Autodesk Inventor part; units mm, degrees
(part 3 of 3)
  spline S181 degree 2 poles (565.5506, -57.2741) (560.0725, -57.2741) (552.7403, -57.9484) (549.8748, -59.044) knots 0 0 0 1 2 2 2
  spline S182 degree 2 poles (549.8748, -59.044) (547.1779, -60.0553) (544.2702, -63.8058) (544.2702, -66.8398) knots 0 0 0 1 2 2 2
  spline S183 degree 2 poles (544.2702, -66.8398) (544.2702, -69.7053) (547.0093, -73.4557) (549.7484, -74.5092) knots 0 0 0 1 2 2 2
  spline S184 degree 2 poles (556.4485, -145.3033) (552.4453, -145.3033) (545.6608, -142.6485) (543.3853, -140.4152) knots 0 0 0 1 2 2 2
  spline S185 degree 2 poles (543.3853, -140.4152) (540.9834, -138.0975) (538.4971, -132.2822) (538.4971, -128.7847) knots 0 0 0 1 2 2 2
  spline S186 degree 2 poles (538.4971, -128.7847) (538.4971, -125.2871) (540.857, -119.514) (543.2168, -117.3228) knots 0 0 0 1 2 2 2
  spline S187 degree 2 poles (543.2168, -117.3228) (546.0401, -114.6258) (555.5215, -111.5918) (562.4323, -111.5918) knots 0 0 0 1 2 2 2
  spline S188 degree 2 poles (562.4323, -111.5918) (569.2168, -111.5918) (580.1309, -114.373) (584.1762, -117.2806) knots 0 0 0 1 2 2 2
  spline S189 degree 2 poles (584.1762, -117.2806) (588.1373, -120.104) (592.562, -129.0375) (592.562, -134.8949) knots 0 0 0 1 2 2 2
  spline S190 degree 2 poles (592.562, -134.8949) (592.562, -136.6226) (592.2249, -139.6566) (591.8456, -140.7944) knots 0 0 0 1 2 2 2
  line L106 (591.8456, -140.7944) -> (585.1454, -140.7944)
  line L107 (585.1454, -140.7944) -> (585.1454, -140.4994)
  spline S191 degree 2 poles (585.1454, -140.4994) (585.6511, -139.5302) (586.536, -135.9905) (586.536, -133.9678) knots 0 0 0 1 2 2 2
  spline S192 degree 2 poles (586.536, -133.9678) (586.536, -127.4784) (577.7711, -119.514) (569.1746, -118.7555) knots 0 0 0 1 2 2 2
  spline S193 degree 2 poles (569.1746, -118.7555) (570.9023, -121.2417) (572.7986, -126.467) (572.7986, -129.5853) knots 0 0 0 1 2 2 2
  spline S194 degree 2 poles (572.7986, -129.5853) (572.7986, -132.6194) (571.5766, -137.1704) (569.7224, -139.6566) knots 0 0 0 1 2 2 2
  spline S195 degree 2 poles (569.7224, -139.6566) (567.5733, -142.5221) (560.9153, -145.3033) (556.4485, -145.3033) knots 0 0 0 1 2 2 2
  spline S196 degree 2 poles (556.1535, -138.2239) (559.3561, -138.2239) (563.6965, -136.5383) (565.2135, -134.6842) knots 0 0 0 1 2 2 2
  spline S197 degree 2 poles (565.2135, -134.6842) (566.3091, -133.2936) (567.0255, -129.8382) (567.0255, -128.0262) knots 0 0 0 1 2 2 2
  spline S198 degree 2 poles (567.0255, -128.0262) (567.0255, -125.5821) (565.5506, -120.9889) (564.16, -118.7555) knots 0 0 0 1 2 2 2
  spline S199 degree 2 poles (564.16, -118.7555) (563.4015, -118.7134) (561.9688, -118.6291) (560.8732, -118.6291) knots 0 0 0 1 2 2 2
  spline S200 degree 2 poles (560.8732, -118.6291) (555.4793, -118.6291) (548.8634, -120.7361) (547.1357, -122.3374) knots 0 0 0 1 2 2 2
  spline S201 degree 2 poles (547.1357, -122.3374) (545.4923, -123.8122) (544.186, -127.0148) (544.186, -128.8268) knots 0 0 0 1 2 2 2
  spline S202 degree 2 poles (544.186, -128.8268) (544.186, -133.0408) (550.1698, -138.2239) (556.1535, -138.2239) knots 0 0 0 1 2 2 2
  spline S203 degree 2 poles (565.5928, -183.8187) (551.6025, -183.8187) (538.4971, -175.6858) (538.4971, -167.2158) knots 0 0 0 1 2 2 2
  spline S204 degree 2 poles (538.4971, -167.2158) (538.4971, -158.6194) (551.8553, -150.5707) (565.5506, -150.5707) knots 0 0 0 1 2 2 2
  spline S205 degree 2 poles (565.5506, -150.5707) (579.6252, -150.5707) (592.6463, -158.7036) (592.6463, -167.2158) knots 0 0 0 1 2 2 2
  spline S206 degree 2 poles (592.6463, -167.2158) (592.6463, -175.7701) (579.1617, -183.8187) (565.5928, -183.8187) knots 0 0 0 1 2 2 2
  spline S207 degree 2 poles (549.7484, -174.8852) (552.3189, -175.8965) (560.2411, -176.7393) (565.5928, -176.7393) knots 0 0 0 1 2 2 2
  spline S208 degree 2 poles (565.5928, -176.7393) (570.9445, -176.7393) (578.8245, -175.8965) (581.4793, -174.843) knots 0 0 0 1 2 2 2
  spline S209 degree 2 poles (581.4793, -174.843) (584.1341, -173.7895) (586.8732, -170.1234) (586.8732, -167.2158) knots 0 0 0 1 2 2 2
  spline S210 degree 2 poles (586.8732, -167.2158) (586.8732, -164.3082) (584.1341, -160.5578) (581.395, -159.4622) knots 0 0 0 1 2 2 2
  spline S211 degree 2 poles (581.395, -159.4622) (578.7403, -158.4087) (570.6495, -157.6502) (565.5506, -157.6502) knots 0 0 0 1 2 2 2
  spline S212 degree 2 poles (565.5506, -157.6502) (560.0725, -157.6502) (552.7403, -158.3244) (549.8748, -159.42) knots 0 0 0 1 2 2 2
  spline S213 degree 2 poles (549.8748, -159.42) (547.1779, -160.4314) (544.2702, -164.1818) (544.2702, -167.2158) knots 0 0 0 1 2 2 2
  spline S214 degree 2 poles (544.2702, -167.2158) (544.2702, -170.0813) (547.0093, -173.8317) (549.7484, -174.8852) knots 0 0 0 1 2 2 2
  line L108 (583.797, -245.4686) -> (539.5928, -222.9662)
  line L109 (539.5928, -222.9662) -> (539.5928, -215.5497)
  line L110 (539.5928, -215.5497) -> (585.4826, -239.3163)
  line L111 (585.4826, -239.3163) -> (585.4826, -212.4735)
  line L112 (585.4826, -212.4735) -> (591.5928, -212.4735)
  line L113 (591.5928, -212.4735) -> (591.5928, -245.4686)
  line L114 (591.5928, -245.4686) -> (583.797, -245.4686)
  spline S215 degree 2 poles (565.5928, -284.1947) (551.6025, -284.1947) (538.4971, -276.0618) (538.4971, -267.5918) knots 0 0 0 1 2 2 2
  spline S216 degree 2 poles (538.4971, -267.5918) (538.4971, -258.9954) (551.8553, -250.9468) (565.5506, -250.9468) knots 0 0 0 1 2 2 2
  spline S217 degree 2 poles (565.5506, -250.9468) (579.6252, -250.9468) (592.6463, -259.0797) (592.6463, -267.5918) knots 0 0 0 1 2 2 2
  spline S218 degree 2 poles (592.6463, -267.5918) (592.6463, -276.1461) (579.1617, -284.1947) (565.5928, -284.1947) knots 0 0 0 1 2 2 2
  spline S219 degree 2 poles (549.7484, -275.2612) (552.3189, -276.2725) (560.2411, -277.1153) (565.5928, -277.1153) knots 0 0 0 1 2 2 2
  spline S220 degree 2 poles (565.5928, -277.1153) (570.9445, -277.1153) (578.8245, -276.2725) (581.4793, -275.219) knots 0 0 0 1 2 2 2
  spline S221 degree 2 poles (581.4793, -275.219) (584.1341, -274.1656) (586.8732, -270.4994) (586.8732, -267.5918) knots 0 0 0 1 2 2 2
  spline S222 degree 2 poles (586.8732, -267.5918) (586.8732, -264.6842) (584.1341, -260.9338) (581.395, -259.8382) knots 0 0 0 1 2 2 2
  spline S223 degree 2 poles (581.395, -259.8382) (578.7403, -258.7847) (570.6495, -258.0262) (565.5506, -258.0262) knots 0 0 0 1 2 2 2
  spline S224 degree 2 poles (565.5506, -258.0262) (560.0725, -258.0262) (552.7403, -258.7004) (549.8748, -259.796) knots 0 0 0 1 2 2 2
  spline S225 degree 2 poles (549.8748, -259.796) (547.1779, -260.8074) (544.2702, -264.5578) (544.2702, -267.5918) knots 0 0 0 1 2 2 2
  spline S226 degree 2 poles (544.2702, -267.5918) (544.2702, -270.4573) (547.0093, -274.2077) (549.7484, -275.2612) knots 0 0 0 1 2 2 2
  spline S227 degree 2 poles (538.4129, -328.9046) (538.4129, -325.0278) (540.7305, -318.6647) (542.8796, -316.4314) knots 0 0 0 1 2 2 2
  spline S228 degree 2 poles (542.8796, -316.4314) (544.9866, -314.2401) (550.7176, -311.9646) (553.9623, -311.9646) knots 0 0 0 1 2 2 2
  spline S229 degree 2 poles (553.9623, -311.9646) (558.1762, -311.9646) (565.2557, -316.4735) (567.3626, -320.7717) knots 0 0 0 1 2 2 2
  line L115 (567.3626, -320.7717) -> (567.5733, -320.7717)
  spline S230 degree 2 poles (567.5733, -320.7717) (569.8067, -316.937) (575.1163, -313.2288) (579.0774, -313.2288) knots 0 0 0 1 2 2 2
  spline S231 degree 2 poles (579.0774, -313.2288) (584.9347, -313.2288) (592.7727, -322.078) (592.7727, -328.9046) knots 0 0 0 1 2 2 2
  spline S232 degree 2 poles (592.7727, -328.9046) (592.7727, -335.984) (585.3561, -344.5383) (579.5409, -344.5383) knots 0 0 0 1 2 2 2
  spline S233 degree 2 poles (579.5409, -344.5383) (576.0433, -344.5383) (569.2168, -340.4508) (567.2783, -336.6161) knots 0 0 0 1 2 2 2
  line L116 (567.2783, -336.6161) -> (567.0676, -336.6161)
  spline S234 degree 2 poles (567.0676, -336.6161) (564.9607, -341.1672) (558.8926, -345.8446) (554.0887, -345.8446) knots 0 0 0 1 2 2 2
  spline S235 degree 2 poles (554.0887, -345.8446) (547.4307, -345.8446) (538.4129, -336.1526) (538.4129, -328.9046) knots 0 0 0 1 2 2 2
  spline S236 degree 2 poles (553.4145, -338.6809) (556.6171, -338.6809) (560.4096, -336.1526) (562.348, -332.5707) knots 0 0 0 1 2 2 2
  spline S237 degree 2 poles (562.348, -332.5707) (563.0223, -331.3908) (564.5814, -327.4297) (565.5928, -324.9435) knots 0 0 0 1 2 2 2
  spline S238 degree 2 poles (565.5928, -324.9435) (563.6965, -322.078) (558.0498, -319.0019) (554.468, -319.0019) knots 0 0 0 1 2 2 2
  spline S239 degree 2 poles (554.468, -319.0019) (549.7484, -319.0019) (543.596, -324.6907) (543.596, -328.9889) knots 0 0 0 1 2 2 2
  spline S240 degree 2 poles (543.596, -328.9889) (543.596, -333.3714) (548.8634, -338.6809) (553.4145, -338.6809) knots 0 0 0 1 2 2 2
  spline S241 degree 2 poles (579.4566, -337.7117) (582.9542, -337.7117) (587.6317, -333.0343) (587.6317, -328.8625) knots 0 0 0 1 2 2 2
  spline S242 degree 2 poles (587.6317, -328.8625) (587.6317, -325.0699) (583.4599, -320.2239) (579.878, -320.2239) knots 0 0 0 1 2 2 2
  spline S243 degree 2 poles (579.878, -320.2239) (577.3075, -320.2239) (573.7257, -322.7101) (572.2929, -325.1963) knots 0 0 0 1 2 2 2
  spline S244 degree 2 poles (572.2929, -325.1963) (571.703, -326.2498) (569.6382, -330.7166) (569.0482, -332.5286) knots 0 0 0 1 2 2 2
  spline S245 degree 2 poles (569.0482, -332.5286) (571.3659, -335.5626) (576.2962, -337.7117) (579.4566, -337.7117) knots 0 0 0 1 2 2 2
  spline S246 degree 2 poles (565.5928, -384.5707) (551.6025, -384.5707) (538.4971, -376.4378) (538.4971, -367.9678) knots 0 0 0 1 2 2 2
  spline S247 degree 2 poles (538.4971, -367.9678) (538.4971, -359.3714) (551.8553, -351.3228) (565.5506, -351.3228) knots 0 0 0 1 2 2 2
  spline S248 degree 2 poles (565.5506, -351.3228) (579.6252, -351.3228) (592.6463, -359.4557) (592.6463, -367.9678) knots 0 0 0 1 2 2 2
  spline S249 degree 2 poles (592.6463, -367.9678) (592.6463, -376.5221) (579.1617, -384.5707) (565.5928, -384.5707) knots 0 0 0 1 2 2 2
  spline S250 degree 2 poles (549.7484, -375.6372) (552.3189, -376.6485) (560.2411, -377.4913) (565.5928, -377.4913) knots 0 0 0 1 2 2 2
  spline S251 degree 2 poles (565.5928, -377.4913) (570.9445, -377.4913) (578.8245, -376.6485) (581.4793, -375.595) knots 0 0 0 1 2 2 2
  spline S252 degree 2 poles (581.4793, -375.595) (584.1341, -374.5416) (586.8732, -370.8754) (586.8732, -367.9678) knots 0 0 0 1 2 2 2
  spline S253 degree 2 poles (586.8732, -367.9678) (586.8732, -365.0602) (584.1341, -361.3098) (581.395, -360.2142) knots 0 0 0 1 2 2 2
  spline S254 degree 2 poles (581.395, -360.2142) (578.7403, -359.1607) (570.6495, -358.4022) (565.5506, -358.4022) knots 0 0 0 1 2 2 2
  spline S255 degree 2 poles (565.5506, -358.4022) (560.0725, -358.4022) (552.7403, -359.0764) (549.8748, -360.172) knots 0 0 0 1 2 2 2
  spline S256 degree 2 poles (549.8748, -360.172) (547.1779, -361.1834) (544.2702, -364.9338) (544.2702, -367.9678) knots 0 0 0 1 2 2 2
  spline S257 degree 2 poles (544.2702, -367.9678) (544.2702, -370.8333) (547.0093, -374.5837) (549.7484, -375.6372) knots 0 0 0 1 2 2 2
  spline S258 degree 2 poles (574.6949, -412.1299) (578.6981, -412.1299) (585.3561, -414.7425) (587.7581, -417.0181) knots 0 0 0 1 2 2 2
  spline S259 degree 2 poles (587.7581, -417.0181) (590.0758, -419.1672) (592.6463, -425.4459) (592.6463, -428.6485) knots 0 0 0 1 2 2 2
  spline S260 degree 2 poles (592.6463, -428.6485) (592.6463, -432.2304) (590.2443, -438.0456) (587.9688, -440.1947) knots 0 0 0 1 2 2 2
  spline S261 degree 2 poles (587.9688, -440.1947) (585.1033, -442.8916) (575.8326, -445.8414) (568.7111, -445.8414) knots 0 0 0 1 2 2 2
  spline S262 degree 2 poles (568.7111, -445.8414) (562.2638, -445.8414) (550.7176, -442.9338) (546.8829, -440.1104) knots 0 0 0 1 2 2 2
  spline S263 degree 2 poles (546.8829, -440.1104) (542.8375, -437.1185) (538.5814, -428.6907) (538.5814, -422.5383) knots 0 0 0 1 2 2 2
  spline S264 degree 2 poles (538.5814, -422.5383) (538.5814, -421.1477) (538.8764, -417.9873) (539.2978, -416.6388) knots 0 0 0 1 2 2 2
  line L117 (539.2978, -416.6388) -> (545.998, -416.6388)
  line L118 (545.998, -416.6388) -> (545.998, -416.9759)
  spline S265 degree 2 poles (545.998, -416.9759) (545.4923, -417.8608) (544.6074, -421.5691) (544.6074, -423.4654) knots 0 0 0 1 2 2 2
  spline S266 degree 2 poles (544.6074, -423.4654) (544.6074, -430.292) (553.6252, -438.0877) (561.9688, -438.6356) knots 0 0 0 1 2 2 2
  spline S267 degree 2 poles (561.9688, -438.6356) (560.0725, -435.8544) (558.3448, -430.7976) (558.3448, -427.8057) knots 0 0 0 1 2 2 2
  spline S268 degree 2 poles (558.3448, -427.8057) (558.3448, -424.9403) (559.609, -420.1785) (561.421, -417.7766) knots 0 0 0 1 2 2 2
  spline S269 degree 2 poles (561.421, -417.7766) (563.5701, -414.9954) (570.1017, -412.1299) (574.6949, -412.1299) knots 0 0 0 1 2 2 2
  spline S270 degree 2 poles (570.2702, -438.8041) (575.5377, -438.8041) (582.1957, -436.8657) (584.0077, -435.138) knots 0 0 0 1 2 2 2
  spline S271 degree 2 poles (584.0077, -435.138) (585.6933, -433.621) (586.9574, -430.4605) (586.9574, -428.6064) knots 0 0 0 1 2 2 2
  spline S272 degree 2 poles (586.9574, -428.6064) (586.9574, -424.3082) (580.8051, -419.2093) (574.9899, -419.2093) knots 0 0 0 1 2 2 2
  spline S273 degree 2 poles (574.9899, -419.2093) (571.703, -419.2093) (567.4469, -420.8949) (565.9299, -422.749) knots 0 0 0 1 2 2 2
  spline S274 degree 2 poles (565.9299, -422.749) (564.8343, -424.0975) (564.1179, -427.4265) (564.1179, -429.3649) knots 0 0 0 1 2 2 2
  spline S275 degree 2 poles (564.1179, -429.3649) (564.1179, -431.5983) (565.677, -436.7393) (566.9834, -438.6777) knots 0 0 0 1 2 2 2
  spline S276 degree 2 poles (566.9834, -438.6777) (567.489, -438.7198) (569.2168, -438.8041) (570.2702, -438.8041) knots 0 0 0 1 2 2 2
  spline S277 degree 2 poles (565.5928, -484.9467) (551.6025, -484.9467) (538.4971, -476.8138) (538.4971, -468.3438) knots 0 0 0 1 2 2 2
  spline S278 degree 2 poles (538.4971, -468.3438) (538.4971, -459.7474) (551.8553, -451.6988) (565.5506, -451.6988) knots 0 0 0 1 2 2 2
  spline S279 degree 2 poles (565.5506, -451.6988) (579.6252, -451.6988) (592.6463, -459.8317) (592.6463, -468.3438) knots 0 0 0 1 2 2 2
  spline S280 degree 2 poles (592.6463, -468.3438) (592.6463, -476.8981) (579.1617, -484.9467) (565.5928, -484.9467) knots 0 0 0 1 2 2 2
  spline S281 degree 2 poles (549.7484, -476.0132) (552.3189, -477.0245) (560.2411, -477.8673) (565.5928, -477.8673) knots 0 0 0 1 2 2 2
  spline S282 degree 2 poles (565.5928, -477.8673) (570.9445, -477.8673) (578.8245, -477.0245) (581.4793, -475.9711) knots 0 0 0 1 2 2 2
  spline S283 degree 2 poles (581.4793, -475.9711) (584.1341, -474.9176) (586.8732, -471.2514) (586.8732, -468.3438) knots 0 0 0 1 2 2 2
  spline S284 degree 2 poles (586.8732, -468.3438) (586.8732, -465.4362) (584.1341, -461.6858) (581.395, -460.5902) knots 0 0 0 1 2 2 2
  spline S285 degree 2 poles (581.395, -460.5902) (578.7403, -459.5367) (570.6495, -458.7782) (565.5506, -458.7782) knots 0 0 0 1 2 2 2
  spline S286 degree 2 poles (565.5506, -458.7782) (560.0725, -458.7782) (552.7403, -459.4524) (549.8748, -460.548) knots 0 0 0 1 2 2 2
  spline S287 degree 2 poles (549.8748, -460.548) (547.1779, -461.5594) (544.2702, -465.3098) (544.2702, -468.3438) knots 0 0 0 1 2 2 2
  spline S288 degree 2 poles (544.2702, -468.3438) (544.2702, -471.2093) (547.0093, -474.9597) (549.7484, -476.0132) knots 0 0 0 1 2 2 2
  spline S289 degree 2 poles (441.8635, 560.8836) (441.8635, 574.8739) (449.9964, 587.9792) (458.4664, 587.9792) knots 0 0 0 1 2 2 2
  spline S290 degree 2 poles (458.4664, 587.9792) (467.0628, 587.9792) (475.1114, 574.6211) (475.1114, 560.9258) knots 0 0 0 1 2 2 2
  spline S291 degree 2 poles (475.1114, 560.9258) (475.1114, 546.8512) (466.9785, 533.8301) (458.4664, 533.8301) knots 0 0 0 1 2 2 2
  spline S292 degree 2 poles (458.4664, 533.8301) (449.9121, 533.8301) (441.8635, 547.3147) (441.8635, 560.8836) knots 0 0 0 1 2 2 2
  spline S293 degree 2 poles (450.797, 576.728) (449.7857, 574.1575) (448.9429, 566.2353) (448.9429, 560.8836) knots 0 0 0 1 2 2 2
  spline S294 degree 2 poles (448.9429, 560.8836) (448.9429, 555.5319) (449.7857, 547.6519) (450.8392, 544.9971) knots 0 0 0 1 2 2 2
  spline S295 degree 2 poles (450.8392, 544.9971) (451.8926, 542.3423) (455.5588, 539.6032) (458.4664, 539.6032) knots 0 0 0 1 2 2 2
  spline S296 degree 2 poles (458.4664, 539.6032) (461.374, 539.6032) (465.1244, 542.3423) (466.22, 545.0814) knots 0 0 0 1 2 2 2
  spline S297 degree 2 poles (466.22, 545.0814) (467.2735, 547.7361) (468.032, 555.8269) (468.032, 560.9258) knots 0 0 0 1 2 2 2
  spline S298 degree 2 poles (468.032, 560.9258) (468.032, 566.4039) (467.3578, 573.7361) (466.2622, 576.6016) knots 0 0 0 1 2 2 2
  spline S299 degree 2 poles (466.2622, 576.6016) (465.2508, 579.2985) (461.5004, 582.2061) (458.4664, 582.2061) knots 0 0 0 1 2 2 2
  spline S300 degree 2 poles (458.4664, 582.2061) (455.6009, 582.2061) (451.8505, 579.4671) (450.797, 576.728) knots 0 0 0 1 2 2 2
  line L119 (361.0823, 586.8836) -> (386.4502, 586.8836)
  line L120 (386.4502, 586.8836) -> (386.4502, 581.5741)
  line L121 (386.4502, 581.5741) -> (377.011, 581.5741)
  line L122 (377.011, 581.5741) -> (377.011, 546.7248)
  line L123 (377.011, 546.7248) -> (386.4502, 546.7248)
  line L124 (386.4502, 546.7248) -> (386.4502, 541.963)
  spline S301 degree 2 poles (386.4502, 541.963) (381.0985, 541.963) (376.0417, 538.929) (375.7046, 534.7151) knots 0 0 0 1 2 2 2
  line L125 (375.7046, 534.7151) -> (370.3108, 534.7151)
  line L126 (370.3108, 534.7151) -> (370.3108, 581.5741)
  line L127 (370.3108, 581.5741) -> (361.0823, 581.5741)
  line L128 (361.0823, 581.5741) -> (361.0823, 586.8836)
  spline S302 degree 2 poles (319.1536, 560.8836) (319.1536, 574.8739) (327.2865, 587.9792) (335.7565, 587.9792) knots 0 0 0 1 2 2 2
  spline S303 degree 2 poles (335.7565, 587.9792) (344.3529, 587.9792) (352.4016, 574.6211) (352.4016, 560.9258) knots 0 0 0 1 2 2 2
  spline S304 degree 2 poles (352.4016, 560.9258) (352.4016, 546.8512) (344.2687, 533.8301) (335.7565, 533.8301) knots 0 0 0 1 2 2 2
  spline S305 degree 2 poles (335.7565, 533.8301) (327.2022, 533.8301) (319.1536, 547.3147) (319.1536, 560.8836) knots 0 0 0 1 2 2 2
  spline S306 degree 2 poles (328.0871, 576.728) (327.0758, 574.1575) (326.233, 566.2353) (326.233, 560.8836) knots 0 0 0 1 2 2 2
  spline S307 degree 2 poles (326.233, 560.8836) (326.233, 555.5319) (327.0758, 547.6519) (328.1293, 544.9971) knots 0 0 0 1 2 2 2
  spline S308 degree 2 poles (328.1293, 544.9971) (329.1828, 542.3423) (332.8489, 539.6032) (335.7565, 539.6032) knots 0 0 0 1 2 2 2
  spline S309 degree 2 poles (335.7565, 539.6032) (338.6641, 539.6032) (342.4145, 542.3423) (343.5101, 545.0814) knots 0 0 0 1 2 2 2
  spline S310 degree 2 poles (343.5101, 545.0814) (344.5636, 547.7361) (345.3221, 555.8269) (345.3221, 560.9258) knots 0 0 0 1 2 2 2
  spline S311 degree 2 poles (345.3221, 560.9258) (345.3221, 566.4039) (344.6479, 573.7361) (343.5523, 576.6016) knots 0 0 0 1 2 2 2
  spline S312 degree 2 poles (343.5523, 576.6016) (342.5409, 579.2985) (338.7905, 582.2061) (335.7565, 582.2061) knots 0 0 0 1 2 2 2
  spline S313 degree 2 poles (335.7565, 582.2061) (332.891, 582.2061) (329.1406, 579.4671) (328.0871, 576.728) knots 0 0 0 1 2 2 2
  line L129 (258.0936, 586.8836) -> (290.1617, 586.8836)
  line L130 (290.1617, 586.8836) -> (290.1617, 579.5092)
  spline S314 degree 2 poles (290.1617, 579.5092) (286.7063, 576.2645) (280.5539, 570.2386) (277.6042, 566.9938) knots 0 0 0 1 2 2 2
  spline S315 degree 2 poles (277.6042, 566.9938) (271.6625, 560.4622) (267.3221, 552.6243) (267.3221, 548.4525) knots 0 0 0 1 2 2 2
  spline S316 degree 2 poles (267.3221, 548.4525) (267.3221, 546.2613) (268.6706, 542.9744) (269.8926, 541.9209) knots 0 0 0 1 2 2 2
  spline S317 degree 2 poles (269.8926, 541.9209) (271.1147, 540.8674) (274.3173, 539.8139) (276.2557, 539.8139) knots 0 0 0 1 2 2 2
  spline S318 degree 2 poles (276.2557, 539.8139) (278.1098, 539.8139) (281.9024, 540.741) (283.6301, 541.4574) knots 0 0 0 1 2 2 2
  spline S319 degree 2 poles (283.6301, 541.4574) (285.105, 542.0473) (287.844, 543.7329) (288.6868, 544.3228) knots 0 0 0 1 2 2 2
  line L131 (288.6868, 544.3228) -> (289.0661, 544.3228)
  line L132 (289.0661, 544.3228) -> (289.0661, 536.9063)
  spline S320 degree 2 poles (289.0661, 536.9063) (286.917, 535.8528) (279.2054, 533.788) (275.75, 533.788) knots 0 0 0 1 2 2 2
  spline S321 degree 2 poles (275.75, 533.788) (268.4599, 533.788) (260.2427, 541.4995) (260.2427, 548.0733) knots 0 0 0 1 2 2 2
  spline S322 degree 2 poles (260.2427, 548.0733) (260.2427, 551.1494) (261.6755, 556.2904) (262.9396, 558.4817) knots 0 0 0 1 2 2 2
  spline S323 degree 2 poles (262.9396, 558.4817) (264.2038, 560.7572) (267.87, 565.224) (269.8926, 567.3731) knots 0 0 0 1 2 2 2
  spline S324 degree 2 poles (269.8926, 567.3731) (273.1795, 570.9549) (281.2281, 578.6243) (283.6301, 580.8577) knots 0 0 0 1 2 2 2
  line L133 (283.6301, 580.8577) -> (258.0936, 580.8577)
  line L134 (258.0936, 580.8577) -> (258.0936, 586.8836)
  spline S325 degree 2 poles (218.7776, 560.8836) (218.7776, 574.8739) (226.9105, 587.9792) (235.3805, 587.9792) knots 0 0 0 1 2 2 2
  spline S326 degree 2 poles (235.3805, 587.9792) (243.9769, 587.9792) (252.0255, 574.6211) (252.0255, 560.9258) knots 0 0 0 1 2 2 2
  spline S327 degree 2 poles (252.0255, 560.9258) (252.0255, 546.8512) (243.8926, 533.8301) (235.3805, 533.8301) knots 0 0 0 1 2 2 2
  spline S328 degree 2 poles (235.3805, 533.8301) (226.8262, 533.8301) (218.7776, 547.3147) (218.7776, 560.8836) knots 0 0 0 1 2 2 2
  spline S329 degree 2 poles (227.7111, 576.728) (226.6998, 574.1575) (225.857, 566.2353) (225.857, 560.8836) knots 0 0 0 1 2 2 2
  spline S330 degree 2 poles (225.857, 560.8836) (225.857, 555.5319) (226.6998, 547.6519) (227.7533, 544.9971) knots 0 0 0 1 2 2 2
  spline S331 degree 2 poles (227.7533, 544.9971) (228.8067, 542.3423) (232.4729, 539.6032) (235.3805, 539.6032) knots 0 0 0 1 2 2 2
  spline S332 degree 2 poles (235.3805, 539.6032) (238.2881, 539.6032) (242.0385, 542.3423) (243.1341, 545.0814) knots 0 0 0 1 2 2 2
  spline S333 degree 2 poles (243.1341, 545.0814) (244.1876, 547.7361) (244.9461, 555.8269) (244.9461, 560.9258) knots 0 0 0 1 2 2 2
  spline S334 degree 2 poles (244.9461, 560.9258) (244.9461, 566.4039) (244.2719, 573.7361) (243.1763, 576.6016) knots 0 0 0 1 2 2 2
  spline S335 degree 2 poles (243.1763, 576.6016) (242.1649, 579.2985) (238.4145, 582.2061) (235.3805, 582.2061) knots 0 0 0 1 2 2 2
  spline S336 degree 2 poles (235.3805, 582.2061) (232.515, 582.2061) (228.7646, 579.4671) (227.7111, 576.728) knots 0 0 0 1 2 2 2
  spline S337 degree 2 poles (175.7533, 539.8139) (177.6495, 539.8139) (181.3999, 540.741) (183.2119, 541.4574) knots 0 0 0 1 2 2 2
  spline S338 degree 2 poles (183.2119, 541.4574) (184.8975, 542.1737) (187.3837, 543.6908) (188.3529, 544.365) knots 0 0 0 1 2 2 2
  line L135 (188.3529, 544.365) -> (188.7743, 544.365)
  line L136 (188.7743, 544.365) -> (188.7743, 536.9906)
  spline S339 degree 2 poles (188.7743, 536.9906) (186.4988, 535.7686) (178.703, 533.788) (175.2055, 533.788) knots 0 0 0 1 2 2 2
  spline S340 degree 2 poles (175.2055, 533.788) (171.6657, 533.788) (166.3983, 535.2207) (164.2492, 536.7378) knots 0 0 0 1 2 2 2
  spline S341 degree 2 poles (164.2492, 536.7378) (161.9737, 538.3812) (159.6139, 543.1429) (159.6139, 546.3455) knots 0 0 0 1 2 2 2
  spline S342 degree 2 poles (159.6139, 546.3455) (159.6139, 550.6438) (165.2606, 557.1332) (169.2217, 557.976) knots 0 0 0 1 2 2 2
  line L137 (169.2217, 557.976) -> (169.2217, 558.4817)
  spline S343 degree 2 poles (169.2217, 558.4817) (167.5782, 558.8188) (163.8278, 560.3358) (162.2265, 561.8528) knots 0 0 0 1 2 2 2
  spline S344 degree 2 poles (162.2265, 561.8528) (160.6252, 563.3277) (158.6025, 568.0473) (158.6025, 571.4606) knots 0 0 0 1 2 2 2
  spline S345 degree 2 poles (158.6025, 571.4606) (158.6025, 574.9582) (161.0045, 580.8998) (163.1957, 583.1754) knots 0 0 0 1 2 2 2
  spline S346 degree 2 poles (163.1957, 583.1754) (165.4713, 585.5352) (171.9186, 587.9792) (176.0061, 587.9792) knots 0 0 0 1 2 2 2
  spline S347 degree 2 poles (176.0061, 587.9792) (179.9251, 587.9792) (187.5944, 586.083) (190.2071, 584.7767) knots 0 0 0 1 2 2 2
  line L138 (190.2071, 584.7767) -> (190.2071, 577.4023)
  line L139 (190.2071, 577.4023) -> (189.7014, 577.4023)
  spline S348 degree 2 poles (189.7014, 577.4023) (187.5102, 579.0036) (180.0936, 581.9533) (176.4275, 581.9533) knots 0 0 0 1 2 2 2
  spline S349 degree 2 poles (176.4275, 581.9533) (174.2784, 581.9533) (169.9802, 580.6049) (168.5474, 579.0457) knots 0 0 0 1 2 2 2
  spline S350 degree 2 poles (168.5474, 579.0457) (167.1568, 577.4865) (165.682, 573.7783) (165.682, 570.9549) knots 0 0 0 1 2 2 2
  spline S351 degree 2 poles (165.682, 570.9549) (165.682, 568.1316) (167.3254, 564.4655) (168.8003, 563.412) knots 0 0 0 1 2 2 2
  spline S352 degree 2 poles (168.8003, 563.412) (170.2751, 562.3585) (174.2784, 561.5579) (176.6382, 561.5579) knots 0 0 0 1 2 2 2
  line L140 (176.6382, 561.5579) -> (179.5879, 561.5579)
  line L141 (179.5879, 561.5579) -> (179.5879, 555.7848)
  line L142 (179.5879, 555.7848) -> (177.2703, 555.7848)
  spline S353 degree 2 poles (177.2703, 555.7848) (172.5928, 555.7848) (166.6933, 551.318) (166.6933, 547.0619) knots 0 0 0 1 2 2 2
  spline S354 degree 2 poles (166.6933, 547.0619) (166.6933, 545.0814) (168.2103, 542.258) (169.4324, 541.4152) knots 0 0 0 1 2 2 2
  spline S355 degree 2 poles (169.4324, 541.4152) (170.7387, 540.5303) (173.9413, 539.8139) (175.7533, 539.8139) knots 0 0 0 1 2 2 2
  spline S356 degree 2 poles (118.4016, 560.8836) (118.4016, 574.8739) (126.5345, 587.9792) (135.0045, 587.9792) knots 0 0 0 1 2 2 2
  spline S357 degree 2 poles (135.0045, 587.9792) (143.6009, 587.9792) (151.6495, 574.6211) (151.6495, 560.9258) knots 0 0 0 1 2 2 2
  spline S358 degree 2 poles (151.6495, 560.9258) (151.6495, 546.8512) (143.5166, 533.8301) (135.0045, 533.8301) knots 0 0 0 1 2 2 2
  spline S359 degree 2 poles (135.0045, 533.8301) (126.4502, 533.8301) (118.4016, 547.3147) (118.4016, 560.8836) knots 0 0 0 1 2 2 2
  spline S360 degree 2 poles (127.3351, 576.728) (126.3238, 574.1575) (125.481, 566.2353) (125.481, 560.8836) knots 0 0 0 1 2 2 2
  spline S361 degree 2 poles (125.481, 560.8836) (125.481, 555.5319) (126.3238, 547.6519) (127.3773, 544.9971) knots 0 0 0 1 2 2 2
  spline S362 degree 2 poles (127.3773, 544.9971) (128.4307, 542.3423) (132.0969, 539.6032) (135.0045, 539.6032) knots 0 0 0 1 2 2 2
  spline S363 degree 2 poles (135.0045, 539.6032) (137.9121, 539.6032) (141.6625, 542.3423) (142.7581, 545.0814) knots 0 0 0 1 2 2 2
  spline S364 degree 2 poles (142.7581, 545.0814) (143.8116, 547.7361) (144.5701, 555.8269) (144.5701, 560.9258) knots 0 0 0 1 2 2 2
  spline S365 degree 2 poles (144.5701, 560.9258) (144.5701, 566.4039) (143.8959, 573.7361) (142.8003, 576.6016) knots 0 0 0 1 2 2 2
  spline S366 degree 2 poles (142.8003, 576.6016) (141.7889, 579.2985) (138.0385, 582.2061) (135.0045, 582.2061) knots 0 0 0 1 2 2 2
  spline S367 degree 2 poles (135.0045, 582.2061) (132.139, 582.2061) (128.3886, 579.4671) (127.3351, 576.728) knots 0 0 0 1 2 2 2
  line L143 (55.951, 569.0165) -> (62.1455, 569.0165)
  line L144 (62.1455, 569.0165) -> (62.1455, 586.8836)
  line L145 (62.1455, 586.8836) -> (68.8457, 586.8836)
  line L146 (68.8457, 586.8836) -> (68.8457, 569.0165)
  line L147 (68.8457, 569.0165) -> (91.8116, 569.0165)
  line L148 (91.8116, 569.0165) -> (91.8116, 561.6843)
  line L149 (91.8116, 561.6843) -> (68.5507, 534.8836)
  line L150 (68.5507, 534.8836) -> (62.1455, 534.8836)
  line L151 (62.1455, 534.8836) -> (62.1455, 563.412)
  line L152 (62.1455, 563.412) -> (55.951, 563.412)
  line L153 (55.951, 563.412) -> (55.951, 569.0165)
  line L154 (68.8457, 563.412) -> (68.8457, 543.1008)
  line L155 (68.8457, 543.1008) -> (86.3335, 563.412)
  line L156 (86.3335, 563.412) -> (68.8457, 563.412)
  spline S368 degree 2 poles (18.0256, 560.8836) (18.0256, 574.8739) (26.1585, 587.9792) (34.6285, 587.9792) knots 0 0 0 1 2 2 2
  spline S369 degree 2 poles (34.6285, 587.9792) (43.2249, 587.9792) (51.2735, 574.6211) (51.2735, 560.9258) knots 0 0 0 1 2 2 2
  spline S370 degree 2 poles (51.2735, 560.9258) (51.2735, 546.8512) (43.1406, 533.8301) (34.6285, 533.8301) knots 0 0 0 1 2 2 2
  spline S371 degree 2 poles (34.6285, 533.8301) (26.0742, 533.8301) (18.0256, 547.3147) (18.0256, 560.8836) knots 0 0 0 1 2 2 2
  spline S372 degree 2 poles (26.9591, 576.728) (25.9478, 574.1575) (25.105, 566.2353) (25.105, 560.8836) knots 0 0 0 1 2 2 2
  spline S373 degree 2 poles (25.105, 560.8836) (25.105, 555.5319) (25.9478, 547.6519) (27.0012, 544.9971) knots 0 0 0 1 2 2 2
  spline S374 degree 2 poles (27.0012, 544.9971) (28.0547, 542.3423) (31.7209, 539.6032) (34.6285, 539.6032) knots 0 0 0 1 2 2 2
  spline S375 degree 2 poles (34.6285, 539.6032) (37.5361, 539.6032) (41.2865, 542.3423) (42.3821, 545.0814) knots 0 0 0 1 2 2 2
  spline S376 degree 2 poles (42.3821, 545.0814) (43.4356, 547.7361) (44.1941, 555.8269) (44.1941, 560.9258) knots 0 0 0 1 2 2 2
  spline S377 degree 2 poles (44.1941, 560.9258) (44.1941, 566.4039) (43.5199, 573.7361) (42.4243, 576.6016) knots 0 0 0 1 2 2 2
  spline S378 degree 2 poles (42.4243, 576.6016) (41.4129, 579.2985) (37.6625, 582.2061) (34.6285, 582.2061) knots 0 0 0 1 2 2 2
  spline S379 degree 2 poles (34.6285, 582.2061) (31.763, 582.2061) (28.0126, 579.4671) (26.9591, 576.728) knots 0 0 0 1 2 2 2
  spline S380 degree 2 poles (-42.4866, 570.365) (-42.4866, 574.1154) (-40.0847, 580.5206) (-37.8934, 582.8804) knots 0 0 0 1 2 2 2
  spline S381 degree 2 poles (-37.8934, 582.8804) (-35.7022, 585.2402) (-29.1706, 587.9792) (-25.1252, 587.9792) knots 0 0 0 1 2 2 2
  spline S382 degree 2 poles (-25.1252, 587.9792) (-21.4169, 587.9792) (-14.1689, 586.3358) (-11.5142, 585.0295) knots 0 0 0 1 2 2 2
  line L157 (-11.5142, 585.0295) -> (-11.5142, 577.6551)
  line L158 (-11.5142, 577.6551) -> (-12.0198, 577.6551)
  spline S383 degree 2 poles (-12.0198, 577.6551) (-12.8205, 578.245) (-15.8124, 579.7621) (-17.6244, 580.4363) knots 0 0 0 1 2 2 2
  spline S384 degree 2 poles (-17.6244, 580.4363) (-19.6892, 581.1527) (-23.1025, 581.9533) (-25.2516, 581.9533) knots 0 0 0 1 2 2 2
  spline S385 degree 2 poles (-25.2516, 581.9533) (-27.3586, 581.9533) (-31.3197, 580.4363) (-32.7524, 578.7929) knots 0 0 0 1 2 2 2
  spline S386 degree 2 poles (-32.7524, 578.7929) (-34.0587, 577.2337) (-35.4072, 573.104) (-35.4072, 570.3228) knots 0 0 0 1 2 2 2
  spline S387 degree 2 poles (-35.4072, 570.3228) (-35.4072, 567.5416) (-33.8902, 564.0019) (-32.4574, 562.822) knots 0 0 0 1 2 2 2
  spline S388 degree 2 poles (-32.4574, 562.822) (-30.9825, 561.5157) (-26.6001, 560.4201) (-23.9453, 560.4201) knots 0 0 0 1 2 2 2
  spline S389 degree 2 poles (-23.9453, 560.4201) (-21.0798, 560.4201) (-15.391, 561.305) (-13.6633, 561.6843) knots 0 0 0 1 2 2 2
  line L159 (-13.6633, 561.6843) -> (-13.6633, 534.8836)
  line L160 (-13.6633, 534.8836) -> (-42.1916, 534.8836)
  line L161 (-42.1916, 534.8836) -> (-42.1916, 540.9938)
  line L162 (-42.1916, 540.9938) -> (-20.3634, 540.9938)
  line L163 (-20.3634, 540.9938) -> (-20.3634, 554.8577)
  spline S390 degree 2 poles (-20.3634, 554.8577) (-21.6276, 554.6891) (-24.0717, 554.5627) (-25.083, 554.5627) knots 0 0 0 1 2 2 2
  spline S391 degree 2 poles (-25.083, 554.5627) (-29.0863, 554.5627) (-34.6065, 555.869) (-37.1349, 557.8074) knots 0 0 0 1 2 2 2
  spline S392 degree 2 poles (-37.1349, 557.8074) (-39.7054, 559.7459) (-42.4866, 565.6454) (-42.4866, 570.365) knots 0 0 0 1 2 2 2
  spline S393 degree 2 poles (-82.3505, 560.8836) (-82.3505, 574.8739) (-74.2176, 587.9792) (-65.7475, 587.9792) knots 0 0 0 1 2 2 2
  spline S394 degree 2 poles (-65.7475, 587.9792) (-57.1511, 587.9792) (-49.1025, 574.6211) (-49.1025, 560.9258) knots 0 0 0 1 2 2 2
  spline S395 degree 2 poles (-49.1025, 560.9258) (-49.1025, 546.8512) (-57.2354, 533.8301) (-65.7475, 533.8301) knots 0 0 0 1 2 2 2
  spline S396 degree 2 poles (-65.7475, 533.8301) (-74.3018, 533.8301) (-82.3505, 547.3147) (-82.3505, 560.8836) knots 0 0 0 1 2 2 2
  spline S397 degree 2 poles (-73.4169, 576.728) (-74.4282, 574.1575) (-75.271, 566.2353) (-75.271, 560.8836) knots 0 0 0 1 2 2 2
  spline S398 degree 2 poles (-75.271, 560.8836) (-75.271, 555.5319) (-74.4282, 547.6519) (-73.3748, 544.9971) knots 0 0 0 1 2 2 2
  spline S399 degree 2 poles (-73.3748, 544.9971) (-72.3213, 542.3423) (-68.6552, 539.6032) (-65.7475, 539.6032) knots 0 0 0 1 2 2 2
  spline S400 degree 2 poles (-65.7475, 539.6032) (-62.8399, 539.6032) (-59.0895, 542.3423) (-57.9939, 545.0814) knots 0 0 0 1 2 2 2
  spline S401 degree 2 poles (-57.9939, 545.0814) (-56.9404, 547.7361) (-56.1819, 555.8269) (-56.1819, 560.9258) knots 0 0 0 1 2 2 2
  spline S402 degree 2 poles (-56.1819, 560.9258) (-56.1819, 566.4039) (-56.8561, 573.7361) (-57.9518, 576.6016) knots 0 0 0 1 2 2 2
  spline S403 degree 2 poles (-57.9518, 576.6016) (-58.9631, 579.2985) (-62.7135, 582.2061) (-65.7475, 582.2061) knots 0 0 0 1 2 2 2
  spline S404 degree 2 poles (-65.7475, 582.2061) (-68.613, 582.2061) (-72.3634, 579.4671) (-73.4169, 576.728) knots 0 0 0 1 2 2 2
  spline S405 degree 2 poles (-144.2111, 570.0279) (-144.2111, 574.0311) (-141.5563, 580.8156) (-139.3229, 583.0911) knots 0 0 0 1 2 2 2
  spline S406 degree 2 poles (-139.3229, 583.0911) (-137.0052, 585.493) (-131.19, 587.9792) (-127.6924, 587.9792) knots 0 0 0 1 2 2 2
  spline S407 degree 2 poles (-127.6924, 587.9792) (-124.1949, 587.9792) (-118.4218, 585.6194) (-116.2305, 583.2596) knots 0 0 0 1 2 2 2
  spline S408 degree 2 poles (-116.2305, 583.2596) (-113.5336, 580.4363) (-110.4996, 570.9549) (-110.4996, 564.0441) knots 0 0 0 1 2 2 2
  spline S409 degree 2 poles (-110.4996, 564.0441) (-110.4996, 557.2596) (-113.2808, 546.3455) (-116.1884, 542.3002) knots 0 0 0 1 2 2 2
  spline S410 degree 2 poles (-116.1884, 542.3002) (-119.0117, 538.3391) (-127.9453, 533.9144) (-133.8026, 533.9144) knots 0 0 0 1 2 2 2
  spline S411 degree 2 poles (-133.8026, 533.9144) (-135.5304, 533.9144) (-138.5644, 534.2515) (-139.7022, 534.6308) knots 0 0 0 1 2 2 2
  line L164 (-139.7022, 534.6308) -> (-139.7022, 541.3309)
  line L165 (-139.7022, 541.3309) -> (-139.4072, 541.3309)
  spline S412 degree 2 poles (-139.4072, 541.3309) (-138.438, 540.8253) (-134.8983, 539.9403) (-132.8756, 539.9403) knots 0 0 0 1 2 2 2
  spline S413 degree 2 poles (-132.8756, 539.9403) (-126.3861, 539.9403) (-118.4218, 548.7053) (-117.6633, 557.3018) knots 0 0 0 1 2 2 2
  spline S414 degree 2 poles (-117.6633, 557.3018) (-120.1495, 555.5741) (-125.3748, 553.6778) (-128.4931, 553.6778) knots 0 0 0 1 2 2 2
  spline S415 degree 2 poles (-128.4931, 553.6778) (-131.5271, 553.6778) (-136.0782, 554.8998) (-138.5644, 556.754) knots 0 0 0 1 2 2 2
  spline S416 degree 2 poles (-138.5644, 556.754) (-141.4299, 558.9031) (-144.2111, 565.5611) (-144.2111, 570.0279) knots 0 0 0 1 2 2 2
  spline S417 degree 2 poles (-137.1317, 570.3228) (-137.1317, 567.1203) (-135.4461, 562.7799) (-133.5919, 561.2629) knots 0 0 0 1 2 2 2
  spline S418 degree 2 poles (-133.5919, 561.2629) (-132.2013, 560.1673) (-128.7459, 559.4509) (-126.9339, 559.4509) knots 0 0 0 1 2 2 2
  spline S419 degree 2 poles (-126.9339, 559.4509) (-124.4898, 559.4509) (-119.8966, 560.9258) (-117.6633, 562.3164) knots 0 0 0 1 2 2 2
  spline S420 degree 2 poles (-117.6633, 562.3164) (-117.6211, 563.0749) (-117.5368, 564.5076) (-117.5368, 565.6032) knots 0 0 0 1 2 2 2
  spline S421 degree 2 poles (-117.5368, 565.6032) (-117.5368, 570.9971) (-119.6438, 577.613) (-121.2451, 579.3407) knots 0 0 0 1 2 2 2
  spline S422 degree 2 poles (-121.2451, 579.3407) (-122.72, 580.9841) (-125.9226, 582.2904) (-127.7346, 582.2904) knots 0 0 0 1 2 2 2
  spline S423 degree 2 poles (-127.7346, 582.2904) (-131.9485, 582.2904) (-137.1317, 576.3066) (-137.1317, 570.3228) knots 0 0 0 1 2 2 2
  spline S424 degree 2 poles (-182.7265, 560.8836) (-182.7265, 574.8739) (-174.5936, 587.9792) (-166.1235, 587.9792) knots 0 0 0 1 2 2 2
  spline S425 degree 2 poles (-166.1235, 587.9792) (-157.5271, 587.9792) (-149.4785, 574.6211) (-149.4785, 560.9258) knots 0 0 0 1 2 2 2
  spline S426 degree 2 poles (-149.4785, 560.9258) (-149.4785, 546.8512) (-157.6114, 533.8301) (-166.1235, 533.8301) knots 0 0 0 1 2 2 2
  spline S427 degree 2 poles (-166.1235, 533.8301) (-174.6778, 533.8301) (-182.7265, 547.3147) (-182.7265, 560.8836) knots 0 0 0 1 2 2 2
  spline S428 degree 2 poles (-173.7929, 576.728) (-174.8043, 574.1575) (-175.647, 566.2353) (-175.647, 560.8836) knots 0 0 0 1 2 2 2
  spline S429 degree 2 poles (-175.647, 560.8836) (-175.647, 555.5319) (-174.8043, 547.6519) (-173.7508, 544.9971) knots 0 0 0 1 2 2 2
  spline S430 degree 2 poles (-173.7508, 544.9971) (-172.6973, 542.3423) (-169.0312, 539.6032) (-166.1235, 539.6032) knots 0 0 0 1 2 2 2
  spline S431 degree 2 poles (-166.1235, 539.6032) (-163.2159, 539.6032) (-159.4655, 542.3423) (-158.3699, 545.0814) knots 0 0 0 1 2 2 2
  spline S432 degree 2 poles (-158.3699, 545.0814) (-157.3164, 547.7361) (-156.5579, 555.8269) (-156.5579, 560.9258) knots 0 0 0 1 2 2 2
  spline S433 degree 2 poles (-156.5579, 560.9258) (-156.5579, 566.4039) (-157.2321, 573.7361) (-158.3278, 576.6016) knots 0 0 0 1 2 2 2
  spline S434 degree 2 poles (-158.3278, 576.6016) (-159.3391, 579.2985) (-163.0895, 582.2061) (-166.1235, 582.2061) knots 0 0 0 1 2 2 2
  spline S435 degree 2 poles (-166.1235, 582.2061) (-168.989, 582.2061) (-172.7394, 579.4671) (-173.7929, 576.728) knots 0 0 0 1 2 2 2
  line L166 (-244.3764, 542.6794) -> (-221.8739, 586.8836)
  line L167 (-221.8739, 586.8836) -> (-214.4574, 586.8836)
  line L168 (-214.4574, 586.8836) -> (-238.224, 540.9938)
  line L169 (-238.224, 540.9938) -> (-211.3812, 540.9938)
  line L170 (-211.3812, 540.9938) -> (-211.3812, 534.8836)
  line L171 (-211.3812, 534.8836) -> (-244.3764, 534.8836)
  line L172 (-244.3764, 534.8836) -> (-244.3764, 542.6794)
  spline S436 degree 2 poles (-283.1025, 560.8836) (-283.1025, 574.8739) (-274.9696, 587.9792) (-266.4996, 587.9792) knots 0 0 0 1 2 2 2
  spline S437 degree 2 poles (-266.4996, 587.9792) (-257.9031, 587.9792) (-249.8545, 574.6211) (-249.8545, 560.9258) knots 0 0 0 1 2 2 2
  spline S438 degree 2 poles (-249.8545, 560.9258) (-249.8545, 546.8512) (-257.9874, 533.8301) (-266.4996, 533.8301) knots 0 0 0 1 2 2 2
  spline S439 degree 2 poles (-266.4996, 533.8301) (-275.0539, 533.8301) (-283.1025, 547.3147) (-283.1025, 560.8836) knots 0 0 0 1 2 2 2
  spline S440 degree 2 poles (-274.1689, 576.728) (-275.1803, 574.1575) (-276.0231, 566.2353) (-276.0231, 560.8836) knots 0 0 0 1 2 2 2
  spline S441 degree 2 poles (-276.0231, 560.8836) (-276.0231, 555.5319) (-275.1803, 547.6519) (-274.1268, 544.9971) knots 0 0 0 1 2 2 2
  spline S442 degree 2 poles (-274.1268, 544.9971) (-273.0733, 542.3423) (-269.4072, 539.6032) (-266.4996, 539.6032) knots 0 0 0 1 2 2 2
  spline S443 degree 2 poles (-266.4996, 539.6032) (-263.5919, 539.6032) (-259.8415, 542.3423) (-258.7459, 545.0814) knots 0 0 0 1 2 2 2
  spline S444 degree 2 poles (-258.7459, 545.0814) (-257.6924, 547.7361) (-256.9339, 555.8269) (-256.9339, 560.9258) knots 0 0 0 1 2 2 2
  spline S445 degree 2 poles (-256.9339, 560.9258) (-256.9339, 566.4039) (-257.6081, 573.7361) (-258.7038, 576.6016) knots 0 0 0 1 2 2 2
  spline S446 degree 2 poles (-258.7038, 576.6016) (-259.7151, 579.2985) (-263.4655, 582.2061) (-266.4996, 582.2061) knots 0 0 0 1 2 2 2
  spline S447 degree 2 poles (-266.4996, 582.2061) (-269.365, 582.2061) (-273.1154, 579.4671) (-274.1689, 576.728) knots 0 0 0 1 2 2 2
  spline S448 degree 2 poles (-327.8124, 588.0635) (-323.9355, 588.0635) (-317.5725, 585.7459) (-315.3391, 583.5967) knots 0 0 0 1 2 2 2
  spline S449 degree 2 poles (-315.3391, 583.5967) (-313.1479, 581.4898) (-310.8723, 575.7588) (-310.8723, 572.5141) knots 0 0 0 1 2 2 2
  spline S450 degree 2 poles (-310.8723, 572.5141) (-310.8723, 568.3002) (-315.3812, 561.2207) (-319.6795, 559.1138) knots 0 0 0 1 2 2 2
  line L173 (-319.6795, 559.1138) -> (-319.6795, 558.9031)
  spline S451 degree 2 poles (-319.6795, 558.9031) (-315.8448, 556.6697) (-312.1365, 551.3601) (-312.1365, 547.399) knots 0 0 0 1 2 2 2
  spline S452 degree 2 poles (-312.1365, 547.399) (-312.1365, 541.5416) (-320.9858, 533.7037) (-327.8124, 533.7037) knots 0 0 0 1 2 2 2
  spline S453 degree 2 poles (-327.8124, 533.7037) (-334.8918, 533.7037) (-343.4461, 541.1203) (-343.4461, 546.9355) knots 0 0 0 1 2 2 2
  spline S454 degree 2 poles (-343.4461, 546.9355) (-343.4461, 550.4331) (-339.3585, 557.2596) (-335.5239, 559.198) knots 0 0 0 1 2 2 2
  line L174 (-335.5239, 559.198) -> (-335.5239, 559.4087)
  spline S455 degree 2 poles (-335.5239, 559.4087) (-340.0749, 561.5157) (-344.7524, 567.5838) (-344.7524, 572.3877) knots 0 0 0 1 2 2 2
  spline S456 degree 2 poles (-344.7524, 572.3877) (-344.7524, 579.0457) (-335.0603, 588.0635) (-327.8124, 588.0635) knots 0 0 0 1 2 2 2
  spline S457 degree 2 poles (-337.5887, 573.0619) (-337.5887, 569.8593) (-335.0603, 566.0668) (-331.4785, 564.1284) knots 0 0 0 1 2 2 2
  spline S458 degree 2 poles (-331.4785, 564.1284) (-330.2986, 563.4541) (-326.3375, 561.895) (-323.8513, 560.8836) knots 0 0 0 1 2 2 2
  spline S459 degree 2 poles (-323.8513, 560.8836) (-320.9858, 562.7799) (-317.9096, 568.4266) (-317.9096, 572.0084) knots 0 0 0 1 2 2 2
  spline S460 degree 2 poles (-317.9096, 572.0084) (-317.9096, 576.728) (-323.5984, 582.8804) (-327.8966, 582.8804) knots 0 0 0 1 2 2 2
  spline S461 degree 2 poles (-327.8966, 582.8804) (-332.2791, 582.8804) (-337.5887, 577.613) (-337.5887, 573.0619) knots 0 0 0 1 2 2 2
  spline S462 degree 2 poles (-336.6195, 547.0198) (-336.6195, 543.5222) (-331.942, 538.8447) (-327.7702, 538.8447) knots 0 0 0 1 2 2 2
  spline S463 degree 2 poles (-327.7702, 538.8447) (-323.9777, 538.8447) (-319.1316, 543.0165) (-319.1316, 546.5984) knots 0 0 0 1 2 2 2
  spline S464 degree 2 poles (-319.1316, 546.5984) (-319.1316, 549.1689) (-321.6179, 552.7507) (-324.1041, 554.1835) knots 0 0 0 1 2 2 2
  spline S465 degree 2 poles (-324.1041, 554.1835) (-325.1576, 554.7734) (-329.6244, 556.8382) (-331.4363, 557.4282) knots 0 0 0 1 2 2 2
  spline S466 degree 2 poles (-331.4363, 557.4282) (-334.4704, 555.1105) (-336.6195, 550.1802) (-336.6195, 547.0198) knots 0 0 0 1 2 2 2
  spline S467 degree 2 poles (-383.4785, 560.8836) (-383.4785, 574.8739) (-375.3456, 587.9792) (-366.8756, 587.9792) knots 0 0 0 1 2 2 2
  spline S468 degree 2 poles (-366.8756, 587.9792) (-358.2791, 587.9792) (-350.2305, 574.6211) (-350.2305, 560.9258) knots 0 0 0 1 2 2 2
  spline S469 degree 2 poles (-350.2305, 560.9258) (-350.2305, 546.8512) (-358.3634, 533.8301) (-366.8756, 533.8301) knots 0 0 0 1 2 2 2
  spline S470 degree 2 poles (-366.8756, 533.8301) (-375.4299, 533.8301) (-383.4785, 547.3147) (-383.4785, 560.8836) knots 0 0 0 1 2 2 2
  spline S471 degree 2 poles (-374.5449, 576.728) (-375.5563, 574.1575) (-376.3991, 566.2353) (-376.3991, 560.8836) knots 0 0 0 1 2 2 2
  spline S472 degree 2 poles (-376.3991, 560.8836) (-376.3991, 555.5319) (-375.5563, 547.6519) (-374.5028, 544.9971) knots 0 0 0 1 2 2 2
  spline S473 degree 2 poles (-374.5028, 544.9971) (-373.4493, 542.3423) (-369.7832, 539.6032) (-366.8756, 539.6032) knots 0 0 0 1 2 2 2
  spline S474 degree 2 poles (-366.8756, 539.6032) (-363.9679, 539.6032) (-360.2175, 542.3423) (-359.1219, 545.0814) knots 0 0 0 1 2 2 2
  spline S475 degree 2 poles (-359.1219, 545.0814) (-358.0684, 547.7361) (-357.3099, 555.8269) (-357.3099, 560.9258) knots 0 0 0 1 2 2 2
  spline S476 degree 2 poles (-357.3099, 560.9258) (-357.3099, 566.4039) (-357.9842, 573.7361) (-359.0798, 576.6016) knots 0 0 0 1 2 2 2
  spline S477 degree 2 poles (-359.0798, 576.6016) (-360.0911, 579.2985) (-363.8415, 582.2061) (-366.8756, 582.2061) knots 0 0 0 1 2 2 2
  spline S478 degree 2 poles (-366.8756, 582.2061) (-369.741, 582.2061) (-373.4914, 579.4671) (-374.5449, 576.728) knots 0 0 0 1 2 2 2
  spline S479 degree 2 poles (-411.0376, 551.7815) (-411.0376, 547.7783) (-413.6503, 541.1203) (-415.9258, 538.7183) knots 0 0 0 1 2 2 2
  spline S480 degree 2 poles (-415.9258, 538.7183) (-418.0749, 536.4006) (-424.3537, 533.8301) (-427.5563, 533.8301) knots 0 0 0 1 2 2 2
  spline S481 degree 2 poles (-427.5563, 533.8301) (-431.1381, 533.8301) (-436.9534, 536.2321) (-439.1025, 538.5076) knots 0 0 0 1 2 2 2
  spline S482 degree 2 poles (-439.1025, 538.5076) (-441.7994, 541.3731) (-444.7491, 550.6438) (-444.7491, 557.7653) knots 0 0 0 1 2 2 2
  spline S483 degree 2 poles (-444.7491, 557.7653) (-444.7491, 564.2126) (-441.8415, 575.7588) (-439.0182, 579.5935) knots 0 0 0 1 2 2 2
  spline S484 degree 2 poles (-439.0182, 579.5935) (-436.0263, 583.6389) (-427.5984, 587.895) (-421.4461, 587.895) knots 0 0 0 1 2 2 2
  spline S485 degree 2 poles (-421.4461, 587.895) (-420.0555, 587.895) (-416.895, 587.6) (-415.5466, 587.1786) knots 0 0 0 1 2 2 2
  line L175 (-415.5466, 587.1786) -> (-415.5466, 580.4784)
  line L176 (-415.5466, 580.4784) -> (-415.8837, 580.4784)
  spline S486 degree 2 poles (-415.8837, 580.4784) (-416.7686, 580.9841) (-420.4769, 581.869) (-422.3731, 581.869) knots 0 0 0 1 2 2 2
  spline S487 degree 2 poles (-422.3731, 581.869) (-429.1997, 581.869) (-436.9955, 572.8512) (-437.5433, 564.5076) knots 0 0 0 1 2 2 2
  spline S488 degree 2 poles (-437.5433, 564.5076) (-434.7621, 566.4039) (-429.7054, 568.1316) (-426.7135, 568.1316) knots 0 0 0 1 2 2 2
  spline S489 degree 2 poles (-426.7135, 568.1316) (-423.848, 568.1316) (-419.0863, 566.8674) (-416.6843, 565.0554) knots 0 0 0 1 2 2 2
  spline S490 degree 2 poles (-416.6843, 565.0554) (-413.9031, 562.9063) (-411.0376, 556.3747) (-411.0376, 551.7815) knots 0 0 0 1 2 2 2
  spline S491 degree 2 poles (-437.7119, 556.2062) (-437.7119, 550.9387) (-435.7735, 544.2807) (-434.0457, 542.4687) knots 0 0 0 1 2 2 2
  spline S492 degree 2 poles (-434.0457, 542.4687) (-432.5287, 540.7831) (-429.3683, 539.519) (-427.5141, 539.519) knots 0 0 0 1 2 2 2
  spline S493 degree 2 poles (-427.5141, 539.519) (-423.2159, 539.519) (-418.1171, 545.6713) (-418.1171, 551.4865) knots 0 0 0 1 2 2 2
  spline S494 degree 2 poles (-418.1171, 551.4865) (-418.1171, 554.7734) (-419.8026, 559.0295) (-421.6568, 560.5465) knots 0 0 0 1 2 2 2
  spline S495 degree 2 poles (-421.6568, 560.5465) (-423.0052, 561.6421) (-426.3342, 562.3585) (-428.2726, 562.3585) knots 0 0 0 1 2 2 2
  spline S496 degree 2 poles (-428.2726, 562.3585) (-430.506, 562.3585) (-435.647, 560.7993) (-437.5854, 559.493) knots 0 0 0 1 2 2 2
  spline S497 degree 2 poles (-437.5854, 559.493) (-437.6276, 558.9874) (-437.7119, 557.2596) (-437.7119, 556.2062) knots 0 0 0 1 2 2 2
  spline S498 degree 2 poles (-483.8545, 560.8836) (-483.8545, 574.8739) (-475.7216, 587.9792) (-467.2516, 587.9792) knots 0 0 0 1 2 2 2
  spline S499 degree 2 poles (-467.2516, 587.9792) (-458.6551, 587.9792) (-450.6065, 574.6211) (-450.6065, 560.9258) knots 0 0 0 1 2 2 2
  spline S500 degree 2 poles (-450.6065, 560.9258) (-450.6065, 546.8512) (-458.7394, 533.8301) (-467.2516, 533.8301) knots 0 0 0 1 2 2 2
  spline S501 degree 2 poles (-467.2516, 533.8301) (-475.8059, 533.8301) (-483.8545, 547.3147) (-483.8545, 560.8836) knots 0 0 0 1 2 2 2
  spline S502 degree 2 poles (-474.9209, 576.728) (-475.9323, 574.1575) (-476.7751, 566.2353) (-476.7751, 560.8836) knots 0 0 0 1 2 2 2
  spline S503 degree 2 poles (-476.7751, 560.8836) (-476.7751, 555.5319) (-475.9323, 547.6519) (-474.8788, 544.9971) knots 0 0 0 1 2 2 2
  spline S504 degree 2 poles (-474.8788, 544.9971) (-473.8253, 542.3423) (-470.1592, 539.6032) (-467.2516, 539.6032) knots 0 0 0 1 2 2 2
  spline S505 degree 2 poles (-467.2516, 539.6032) (-464.344, 539.6032) (-460.5936, 542.3423) (-459.4979, 545.0814) knots 0 0 0 1 2 2 2
  spline S506 degree 2 poles (-459.4979, 545.0814) (-458.4444, 547.7361) (-457.6859, 555.8269) (-457.6859, 560.9258) knots 0 0 0 1 2 2 2
  spline S507 degree 2 poles (-457.6859, 560.9258) (-457.6859, 566.4039) (-458.3602, 573.7361) (-459.4558, 576.6016) knots 0 0 0 1 2 2 2
  spline S508 degree 2 poles (-459.4558, 576.6016) (-460.4671, 579.2985) (-464.2175, 582.2061) (-467.2516, 582.2061) knots 0 0 0 1 2 2 2
  spline S509 degree 2 poles (-467.2516, 582.2061) (-470.1171, 582.2061) (-473.8675, 579.4671) (-474.9209, 576.728) knots 0 0 0 1 2 2 2
  point P0 (0, 0)
  constraints: 8 other
extrude "Выдавливание7" add sketch "Эскиз7" against normal blind 0.5 separate body
